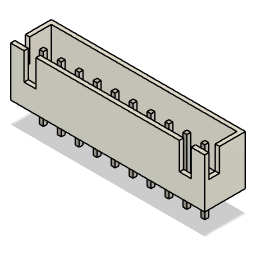
XH 2.54mm 10pin connector (Autodesk Fusion 360 design; units mm, degrees)
Autodesk Fusion 360 part; units mm, degrees
sketch "Sketch1" plane through (0, 0, 0) normal (0, 1, 0) x (1, 0, 0)
  line L0 (13.735, -2.88) -> (-13.735, -2.88)
  line L1 (-13.735, -2.88) -> (-13.735, 2.88)
  line L2 (-13.735, 2.88) -> (13.735, 2.88)
  line L3 (13.735, 2.88) -> (13.735, -2.88)
  line L4 (13.735, -2.88) -> (-13.735, 2.88) construction
  line L5 (-13.735, -2.88) -> (13.735, 2.88) construction
  line L6 (13.135, -2.28) -> (-13.135, -2.28)
  line L7 (-13.135, -2.28) -> (-13.135, 2.28)
  line L8 (-13.135, 2.28) -> (13.135, 2.28)
  line L9 (13.135, 2.28) -> (13.135, -2.28)
  dimension "d1" = 27.47
  dimension "d2" = 5.76
  dimension "d3" = 0.6
  constraint horizontal L0
  constraint perpendicular L0 L1
  constraint parallel L0 L2
  constraint parallel L1 L3
  constraint coincident L4 origin
  constraint coincident L5 origin
  measures "d1" distance of L1.end L2.end
  measures "d2" distance of L0.end L1.end
extrude "Extrude1" add sketch "Sketch1" along normal blind 0.6 contours L6 L7 L8 L9 makes body 1
extrude "Extrude2" add sketch "Sketch1" along normal blind 7 bodies 1
sketch "Sketch2" plane through (0, 0, 2.88) normal (0, 0, 1) x (1, 0, 0)
  line L0 (-13.735, 0) -> (13.735, 0)
  line L1 (13.735, 0) -> (13.735, 7)
  line L2 (13.735, 7) -> (-13.735, 7)
  line L3 (-13.735, 7) -> (-13.735, 0)
  line L4 (13.735, 7) -> (11.835, 7) construction
  line L5 (11.835, 7) -> (11.835, 3.15)
  line L6 (11.835, 3.15) -> (10.155, 3.15)
  line L7 (10.155, 3.15) -> (10.155, 7)
  line L8 (10.155, 3.15) -> (-14.4163, 3.15) construction
  line L9 (-13.735, 3.15) -> (-11.835, 3.15) construction
  line L10 (-11.835, 3.15) -> (-11.835, 7)
  line L11 (-11.835, 3.15) -> (-10.155, 3.15)
  line L12 (-10.155, 3.15) -> (-10.155, 7)
  dimension "d8" = 1.9
  dimension "d9" = 3.85
  dimension "d10" = 1.68
  dimension "d11" = 90
  dimension "d12" = 1.9
  dimension "d13" = 1.68
  dimension "d14" = 90
  constraint coincident L1.end L2.start
  constraint perpendicular L1 L4
  constraint perpendicular L4 L5
  constraint perpendicular L5 L6
  constraint coincident L2 L7.end
  constraint perpendicular L3 L8
  constraint coincident L3 L9.start
  constraint coincident L8 L9.start
  constraint perpendicular L3 L9
  constraint perpendicular L8 L10
  constraint perpendicular L10 L11
  constraint coincident L2 L12.end
  measures "d8" distance of L1.end L4.end
  measures "d9" distance of L4.end L5.end
  measures "d10" distance of L5.end L6.end
  measures "d11" angle of L6 L7
  measures "d12" distance of L9.start L9.end
  measures "d13" distance of L9.end L11.end
  measures "d14" angle of L11 L12
extrude "Extrude3" cut sketch "Sketch2" against normal blind 1 contours L2 L10 L11 L12 | L2 L5 L6 L7 bodies 1
sketch "Sketch3" plane through (13.735, 0, 0) normal (1, 0, 0) x (0, 0, -1)
  line L0 (-2.88, 0) -> (2.88, 0)
  line L1 (2.88, 0) -> (2.88, 7)
  line L2 (2.88, 7) -> (-2.88, 7)
  line L3 (-2.88, 7) -> (-2.88, 0)
  line L4 (-2.88, 7) -> (-2.28, 7) construction
  line L5 (-2.28, 7) -> (-2.28, 3.7)
  line L6 (-2.28, 3.7) -> (-0.78, 3.7)
  line L7 (-0.78, 3.7) -> (-0.78, 7)
  point P0 (-2.28, 7)
  dimension "d17" = 3.3
  dimension "d18" = 1.5
  constraint coincident L2.end L3.start
  constraint coincident P0 L4.end
  constraint perpendicular L4 L5
  constraint perpendicular L5 L6
  constraint perpendicular L6 L7
  measures "d17" distance of P0 L5.end
  measures "d18" distance of L5.end L6.end
extrude "Extrude4" cut sketch "Sketch3" against normal blind 31 contours L2 L5 L6 L7 bodies 1
sketch "Sketch4" plane through (0, 0, 0) normal (0, -1, 0) x (1, 0, 0)
  line L0 (-13.735, -2.88) -> (13.735, -2.88)
  line L1 (13.735, -2.88) -> (13.735, 2.88)
  line L2 (13.735, 2.88) -> (-13.735, 2.88)
  line L3 (-13.735, 2.88) -> (-13.735, -2.88)
  line L4 (13.735, 2.88) -> (13.735, 0.83) construction
  line L5 (13.735, 0.83) -> (-14.1487, 0.83) construction
  line L6 (13.735, -2.88) -> (13.735, 0.28) construction
  line L7 (13.735, 0.28) -> (-14.6727, 0.28) construction
  line L8 (13.735, 0.28) -> (13.735, 0.83) construction
  line L9 (0, 0) -> (0, 0.83) construction
  line L10 (0, 0.83) -> (0, 0.28) construction
  line L11 (0, 0.555) -> (1.27, 0.555) construction
  line L12 (0, 0.555) -> (-1.27, 0.555) construction
  line L13 (1.27, 0.555) -> (3.81, 0.555) construction
  line L14 (3.81, 0.555) -> (6.35, 0.555) construction
  line L15 (6.35, 0.555) -> (8.89, 0.555) construction
  line L16 (8.89, 0.555) -> (11.43, 0.555) construction
  line L17 (11.155, 0.28) -> (11.705, 0.28)
  line L18 (11.705, 0.28) -> (11.705, 0.83)
  line L19 (11.705, 0.83) -> (11.155, 0.83)
  line L20 (11.155, 0.83) -> (11.155, 0.28)
  line L21 (11.155, 0.28) -> (11.705, 0.83) construction
  line L22 (11.705, 0.28) -> (11.155, 0.83) construction
  line L23 (9.165, 0.28) -> (8.615, 0.28)
  line L24 (8.615, 0.28) -> (8.615, 0.83)
  line L25 (8.615, 0.83) -> (9.165, 0.83)
  line L26 (9.165, 0.83) -> (9.165, 0.28)
  line L27 (9.165, 0.28) -> (8.615, 0.83) construction
  line L28 (8.615, 0.28) -> (9.165, 0.83) construction
  line L29 (6.625, 0.83) -> (6.075, 0.83)
  line L30 (6.075, 0.83) -> (6.075, 0.28)
  line L31 (6.075, 0.28) -> (6.625, 0.28)
  line L32 (6.625, 0.28) -> (6.625, 0.83)
  line L33 (6.625, 0.83) -> (6.075, 0.28) construction
  line L34 (6.075, 0.83) -> (6.625, 0.28) construction
  line L35 (4.085, 0.83) -> (3.535, 0.83)
  line L36 (3.535, 0.83) -> (3.535, 0.28)
  line L37 (3.535, 0.28) -> (4.085, 0.28)
  line L38 (4.085, 0.28) -> (4.085, 0.83)
  line L39 (4.085, 0.83) -> (3.535, 0.28) construction
  line L40 (3.535, 0.83) -> (4.085, 0.28) construction
  line L41 (1.545, 0.83) -> (0.995, 0.83)
  line L42 (0.995, 0.83) -> (0.995, 0.28)
  line L43 (0.995, 0.28) -> (1.545, 0.28)
  line L44 (1.545, 0.28) -> (1.545, 0.83)
  line L45 (1.545, 0.83) -> (0.995, 0.28) construction
  line L46 (0.995, 0.83) -> (1.545, 0.28) construction
  line L47 (-1.27, 0.555) -> (-3.81, 0.555) construction
  line L48 (-3.81, 0.555) -> (-6.35, 0.555) construction
  line L49 (-6.35, 0.555) -> (-8.89, 0.555) construction
  line L50 (-8.89, 0.555) -> (-11.43, 0.555) construction
  line L51 (-11.155, 0.28) -> (-11.705, 0.28)
  line L52 (-11.705, 0.28) -> (-11.705, 0.83)
  line L53 (-11.705, 0.83) -> (-11.155, 0.83)
  line L54 (-11.155, 0.83) -> (-11.155, 0.28)
  line L55 (-11.155, 0.28) -> (-11.705, 0.83) construction
  line L56 (-11.705, 0.28) -> (-11.155, 0.83) construction
  line L57 (-8.615, 0.28) -> (-9.165, 0.28)
  line L58 (-9.165, 0.28) -> (-9.165, 0.83)
  line L59 (-9.165, 0.83) -> (-8.615, 0.83)
  line L60 (-8.615, 0.83) -> (-8.615, 0.28)
  line L61 (-8.615, 0.28) -> (-9.165, 0.83) construction
  line L62 (-9.165, 0.28) -> (-8.615, 0.83) construction
  line L63 (-6.075, 0.28) -> (-6.625, 0.28)
  line L64 (-6.625, 0.28) -> (-6.625, 0.83)
  line L65 (-6.625, 0.83) -> (-6.075, 0.83)
  line L66 (-6.075, 0.83) -> (-6.075, 0.28)
  line L67 (-6.075, 0.28) -> (-6.625, 0.83) construction
  line L68 (-6.625, 0.28) -> (-6.075, 0.83) construction
  line L69 (-3.535, 0.28) -> (-4.085, 0.28)
  line L70 (-4.085, 0.28) -> (-4.085, 0.83)
  line L71 (-4.085, 0.83) -> (-3.535, 0.83)
  line L72 (-3.535, 0.83) -> (-3.535, 0.28)
  line L73 (-3.535, 0.28) -> (-4.085, 0.83) construction
  line L74 (-4.085, 0.28) -> (-3.535, 0.83) construction
  line L75 (-0.995, 0.28) -> (-1.545, 0.28)
  line L76 (-1.545, 0.28) -> (-1.545, 0.83)
  line L77 (-1.545, 0.83) -> (-0.995, 0.83)
  line L78 (-0.995, 0.83) -> (-0.995, 0.28)
  line L79 (-0.995, 0.28) -> (-1.545, 0.83) construction
  line L80 (-1.545, 0.28) -> (-0.995, 0.83) construction
  point P0 (11.2775, 0.555)
  point P1 (11.43, 0.555)
  point P2 (8.89, 0.555)
  point P3 (6.35, 0.555)
  point P4 (3.81, 0.555)
  point P5 (1.27, 0.555)
  point P6 (-11.43, 0.555)
  point P7 (-8.89, 0.555)
  point P8 (-6.35, 0.555)
  point P9 (-3.81, 0.555)
  point P10 (-1.27, 0.555)
  dimension "d21" = 2.05
  dimension "d22" = 90
  dimension "d23" = 3.16
  dimension "d25" = 1.27
  dimension "d26" = 1.27
  dimension "d27" = 2.54
  dimension "d28" = 2.54
  dimension "d29" = 2.54
  dimension "d30" = 2.54
  dimension "d31" = 0.55
  dimension "d32" = 0.55
  dimension "d33" = 0.55
  dimension "d34" = 0.55
  dimension "d35" = 0.55
  dimension "d36" = 2.54
  dimension "d37" = 2.54
  dimension "d38" = 2.54
  dimension "d39" = 2.54
  dimension "d40" = 0.55
  dimension "d41" = 0.55
  dimension "d42" = 0.55
  dimension "d43" = 0.55
  dimension "d44" = 0.55
  constraint coincident L1.end L2.start
  constraint perpendicular L2 L4
  constraint coincident L0.end L1.start
  constraint coincident L1 L6.end
  constraint perpendicular L3 L7
  constraint coincident L9.start origin
  constraint coincident L5 L9.end
  constraint perpendicular L5 L9
  constraint coincident L9 L10.end
  constraint coincident L7 L10.end
  constraint midpoint L10 L11.start
  constraint perpendicular L9 L11
  constraint perpendicular L9 L12
  constraint horizontal L13
  constraint parallel L13 L14
  constraint parallel L7 L15
  constraint parallel L15 L16
  constraint horizontal L17
  constraint perpendicular L17 L18
  constraint parallel L17 L19
  constraint parallel L18 L20
  constraint coincident L21 P1
  constraint coincident L22 P1
  constraint coincident P1 L16.end
  constraint horizontal L23
  constraint perpendicular L23 L24
  constraint parallel L23 L25
  constraint parallel L24 L26
  constraint coincident L27 P2
  constraint coincident L28 P2
  constraint coincident P2 L15.end
  constraint horizontal L29
  constraint perpendicular L29 L30
  constraint parallel L29 L31
  constraint parallel L30 L32
  constraint coincident L33 P3
  constraint coincident L34 P3
  constraint coincident P3 L14.end
  constraint horizontal L35
  constraint perpendicular L35 L36
  constraint parallel L35 L37
  constraint parallel L36 L38
  constraint coincident L39 P4
  constraint coincident L40 P4
  constraint coincident P4 L13.end
  constraint horizontal L41
  constraint perpendicular L41 L42
  constraint parallel L41 L43
  constraint parallel L42 L44
  constraint coincident L45 P5
  constraint coincident L46 P5
  constraint coincident P5 L11.end
  constraint parallel L12 L47
  constraint parallel L47 L48
  constraint parallel L48 L49
  constraint parallel L49 L50
  constraint horizontal L51
  constraint perpendicular L51 L52
  constraint parallel L51 L53
  constraint parallel L52 L54
  constraint coincident L55 P6
  constraint coincident L56 P6
  constraint coincident P6 L50.end
  constraint horizontal L57
  constraint perpendicular L57 L58
  constraint parallel L57 L59
  constraint parallel L58 L60
  constraint coincident L61 P7
  constraint coincident L62 P7
  constraint coincident P7 L49.end
  constraint horizontal L63
  constraint perpendicular L63 L64
  constraint parallel L63 L65
  constraint parallel L64 L66
  constraint coincident L67 P8
  constraint coincident L68 P8
  constraint coincident P8 L48.end
  constraint horizontal L69
  constraint perpendicular L69 L70
  constraint parallel L69 L71
  constraint parallel L70 L72
  constraint coincident L73 P9
  constraint coincident L74 P9
  constraint coincident P9 L47.end
  constraint horizontal L75
  constraint perpendicular L75 L76
  constraint parallel L75 L77
  constraint parallel L76 L78
  constraint coincident L79 P10
  constraint coincident L80 P10
  constraint coincident P10 L12.end
  measures "d21" distance of L1.end L4.end
  measures "d22" angle of L4 L5
  measures "d23" distance of L0.end L6.end
  measures "d25" distance of L11.start P5
  measures "d26" distance of L11.start P10
  measures "d27" distance of P5 P4
  measures "d28" distance of P4 P3
  measures "d29" distance of P3 P2
  measures "d30" distance of P2 P1
  measures "d31" distance of L18.end L19.end
  measures "d32" distance of L24.end L25.end
  measures "d33" distance of L30.end L31.end
  measures "d34" distance of L36.end L37.end
  measures "d35" distance of L42.end L43.end
  measures "d36" distance of P10 P9
  measures "d37" distance of P9 P8
  measures "d38" distance of P8 P7
  measures "d39" distance of P7 P6
  measures "d40" distance of L52.end L53.end
  measures "d41" distance of L58.end L59.end
  measures "d42" distance of L64.end L65.end
  measures "d43" distance of L70.end L71.end
  measures "d44" distance of L76.end L77.end
extrude "Extrude5" cut sketch "Sketch4" against normal blind 1.5 contours L17 L18 L19 L20 | L23 L24 L25 L26 | L29 L30 L31 L32 | L35 L36 L37 L38 | L41 L42 L43 L44 | L51 L52 L53 L54 | L57 L58 L59 L60 | L63 L64 L65 L66 | L69 L70 L71 L72 | L75 L76 L77 L78 bodies 1
extrude "Extrude6" add sketch "Sketch4" along normal blind 2.98 and the other way blind 6.2 separate body contours L17 L18 L19 L20 | L23 L24 L25 L26 | L29 L30 L31 L32 | L35 L36 L37 L38 | L41 L42 L43 L44 | L51 L52 L53 L54 | L57 L58 L59 L60 | L63 L64 L65 L66 | L69 L70 L71 L72 | L75 L76 L77 L78 makes body 2 at (-6.075, 0.08, 0.4633) makes body 3 at (4.085, 3.14, 0.4633) makes body 4 at (11.5217, 0.08, 0.28) makes body 5 at (1.545, 3.14, 0.4633) makes body 6 at (-8.615, 0.08, 0.4633) makes body 7 at (-3.9017, 0.08, 0.28) makes body 8 at (6.2583, 3.14, 0.28) makes body 9 at (8.7983, 0.08, 0.28) makes body 10 at (-1.3617, 0.08, 0.28) makes body 11 at (-11.155, 0.08, 0.4633)
